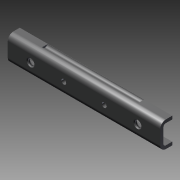
# Autodesk Inventor part: BSPG1560 Rail
Saved by Autodesk Inventor 2016 (Build 200138000, 138)
## iProperties
Category: PARTsolutions
Company: IKO
Created: 2015-05-07
Part Number: BSPG1560 Rail
Catalog Web Link: www.cadenas.de
Description: BSPG- Rail-
Vendor: IKO
Document SubType Name: Modeling
Designer: PARTuser1
Manufacturer: IKO
Mass: 0.912074 g
Surface Area: 19.2322 cm^2
Volume: 0.912074 cm^3
Density: 1 g/cm^3
Material: Generic
Appearance: PSOLRGB-192-192-192
PSOL_IDENT_0: {$CADENAS_DATA\23d-libs\iko\linear_way_series\precise_ball_slide\bspg_3.prj},172 {VTYP=3D},{NB=BSPG1
PSOL_IDENT_1: 560 Rail},{LINA=BSPG1560 Rail},{NN=BSPG- Rail},{DATE=18.01.2008 10:02:28},{GEOMDATE=09.10.2007 06:11
PSOL_IDENT_2: :00},{VERSION=},{LINEID=60},{LINESUBID=-1},{WBVAR=}  {NB=BSPG1560 Rail},{LINA=BSPG1560 Rail},{KT=DUM
PSOL_IDENT_3: MY},{IDNR=},{TP=BSPG},{SZ=15},{W=15.000},{H=8.000},{L=60.000},{MS=40.000},{L1=40.000},{M1=3.000},{S1=
PSOL_IDENT_4: 2.500},{SH1=7.000},{ST1=1.200},{LB=57.000},{SW=9.600},{L2=40.000},{M2=3.000},{S2=3.000},{SH2=4.500},
PSOL_IDENT_5: {ST2=1.200},{R=2.790},{R1=1.300},{W2=5.800},{ST3=2.000},{T1=1.400},{LN=15.100},{DN=1.800},{RR=1.300}
PSOL_IDENT_6: ,{RR1=1.300},{LX=36.000},{DA=2.200},{X=3.000}
SUPPLIER: IKO
ARTICLENO: BSPG1560 Rail
BOMINFO: BSPG1560 Rail
CREATOR: CADENAS GmbH
Title: BSPG1560 Rail
Author: Cadenas PARTsolutions
Autodesk Inventor part; units mm, degrees
sketch "Sketch_1" plane through (0, 0, 0) normal (1, 0, 0) x (0, 1, 0)
  line L0 (4.5, 4.8) -> (2.15, 4.8)
  arc A0 (2.15, 4.8) -> (0, 2.65) centre (2.15, 2.65) ccw
  line L1 (0, 2.65) -> (0, -2.65)
  arc A1 (0, -2.65) -> (2.15, -4.8) centre (2.15, -2.65) ccw
  line L2 (2.15, -4.8) -> (4.5, -4.8)
  line L3 (4.5, -4.8) -> (4.5, -3.6)
  line L4 (4.5, -3.6) -> (2, -3.6)
  arc A2 (1.2, -2.8) -> (2, -3.6) centre (2, -2.8) ccw
  line L5 (1.2, -2.8) -> (1.2, 2.8)
  arc A3 (2, 3.6) -> (1.2, 2.8) centre (2, 2.8) ccw
  line L6 (2, 3.6) -> (4.5, 3.6)
  line L7 (4.5, 3.6) -> (4.5, 4.8)
  constraints: 16 end point, 8 point on circle, 4 centre point
extrude "Extrusion1" add sketch "Sketch_1" along normal blind 57
sketch "Sketch_2" plane through (8.5, 0, 0) normal (1, 0, 0) x (0, 0, -1)
  line L0 (0, 0) -> (0, 1.2)
  line L1 (0, 1.2) -> (1.5, 1.2)
  line L2 (1.5, 1.2) -> (1.2295, 0.9295)
  line L3 (1.2295, 0.9295) -> (1.2295, 0.2705)
  line L4 (1.2295, 0.2705) -> (1.5, 0)
  line L5 (1.5, 0) -> (0, 0)
  line L6 (0, 0) -> (0, 1.2)
  constraints: 14 end point
revolve "Revolution1" cut sketch "Sketch_2" angle 360 about axis through (8.5, 0, 0) along (0, -1, 0)
thread "Thread1" size "M3x0.5" class "6H" standard "ISO Metric profile" full length
sketch "Sketch_3" plane through (48.5, 0, 0) normal (1, 0, 0) x (0, 0, -1)
  line L0 (0, 0) -> (0, 1.2)
  line L1 (0, 1.2) -> (1.5, 1.2)
  line L2 (1.5, 1.2) -> (1.2295, 0.9295)
  line L3 (1.2295, 0.9295) -> (1.2295, 0.2705)
  line L4 (1.2295, 0.2705) -> (1.5, 0)
  line L5 (1.5, 0) -> (0, 0)
  line L6 (0, 0) -> (0, 1.2)
  constraints: 14 end point
revolve "Revolution2" cut sketch "Sketch_3" angle 360 about axis through (48.5, 0, 0) along (0, -1, 0)
thread "Thread2" size "M3x0.5" class "6H" standard "ISO Metric profile" full length
sketch "Sketch4" plane through (0, 0, -2.65) normal (0, -1, 0) x (1, 0, 0)
  point P0 (20.95, 2.65)
hole "Hole1" at (20.95, 0, 0) direction (0, 1, 0) diameter 1.8 depth 1.2
sketch "Sketch5" plane through (0, 0, -2.65) normal (0, -1, 0) x (1, 0, 0)
  point P0 (36.05, 2.65)
hole "Hole2" at (36.05, 0, 0) direction (0, 1, 0) diameter 1.8 depth 1.2
sketch "Sketch_8" plane through (28.5, 0, 0) normal (1, 0, 0) x (0, 0, -1)
  arc A0 (5.1667, 4.4667) -> (5.1667, 2.2667) centre (5.1667, 3.3667) ccw
  line L0 (5.1667, 2.2667) -> (5.1667, 4.4667)
  constraints: 2 end point, 2 point on circle, 1 centre point
extrude "Extrusion2" cut sketch "Sketch_8" along normal mid plane 36
sketch "Sketch_10" plane through (28.5, 0, 0) normal (1, 0, 0) x (0, 0, -1)
  arc A0 (-5.1667, 2.2667) -> (-5.1667, 4.4667) centre (-5.1667, 3.3667) ccw
  line L0 (-5.1667, 4.4667) -> (-5.1667, 2.2667)
  constraints: 2 end point, 2 point on circle, 1 centre point
extrude "Extrusion3" cut sketch "Sketch_10" along normal mid plane 36
ref_plane "bspg_r2_XY" through (28.5, 4.5, 0) normal (1, 0, 0) x (0, 0, -1)
ref_plane "bspg_r2_YZ" through (28.5, 4.5, 0) normal (0, 0, -1) x (0, 1, 0)
ref_plane "bspg_r2_ZX" through (28.5, 4.5, 0) normal (0, 1, 0) x (1, 0, 0)
body "Solid1"
